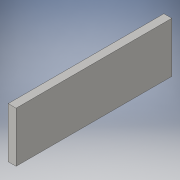
# Autodesk Inventor part: Bread Board
Saved by Autodesk Inventor 2016 (Build 200138000, 138)
## iProperties
Created: 2016-10-05
Part Number: Bread Board
Material: Generic
Document SubType Name: Modeling
Designer: brandn
Density: 1 g/cm^3
Appearance: Default
Author: brandn
Autodesk Inventor part; units mm, degrees
ref_plane "YZ Plane" through (0, 0, 0) normal (1, 0, 0) x (0, 1, 0)
ref_plane "XZ Plane" through (0, 0, 0) normal (0, 1, 0) x (-1, 0, 0)
ref_plane "XY Plane" through (0, 0, 0) normal (0, 0, 1) x (1, 0, 0)
sketch "Sketch1" plane through (0, 0, 0) normal (1, 0, 0) x (0, 1, 0)
  line L0 (33.5033, 76.6496) -> (-20.7003, 76.6496)
  line L1 (-20.7003, 76.6496) -> (-20.7003, -90.9904)
  line L2 (-20.7003, -90.9904) -> (33.5033, -90.9904)
  line L3 (33.5033, -90.9904) -> (33.5033, 76.6496)
  point P0 (0, 0)
  dimension "d0" = 167.64
  dimension "d1" = 54.2036
  constraints: 8 end point, 2 parallel, 1 horizontal, 1 perpendicular
  measures "d0" distance of L2.end L0.start
  measures "d1" distance of L0.start L0.end
extrude "Extrusion1" add sketch "Sketch1" along normal blind 8.509
body "Solid1"
